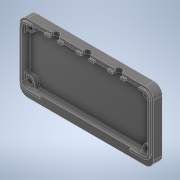
# Autodesk Inventor part: casing-bot
Saved by Autodesk Inventor 2021 (Build 250183000, 183)
## iProperties
Created: 2022-04-08
Part Number: casing-bot
Material: PET Plastic
Document SubType Name: Modeling
Designer: Staňa
Density: 1.541 g/cm^3
Appearance: Smooth - Black
Author: Staňa
Autodesk Inventor part; units mm, degrees
ref_plane "YZ Plane" through (0, 0, 0) normal (1, 0, 0) x (0, 1, 0)
ref_plane "XZ Plane" through (0, 0, 0) normal (0, 1, 0) x (-1, 0, 0)
sketch "Sketch1" plane through (0, 0, 0) normal (0, 0, 1) x (1, 0, 0)
  line L0 (-50, 17.455) -> (-50, -20) construction
  arc A0 (-46.75, 20.705) -> (-50, 17.455) centre (-46.7497, 17.4547) ccw construction
  arc A1 (-50, -20) -> (-46.75, -23.25) centre (-46.7497, -19.9997) ccw construction
  line L1 (-46.75, -23.25) -> (46.75, -23.25) construction
  arc A2 (46.75, -23.25) -> (50, -20) centre (46.7497, -19.9997) ccw construction
  line L2 (50, -20) -> (50, 17.455) construction
  arc A3 (50, 17.455) -> (46.75, 20.705) centre (46.7497, 17.4547) ccw construction
  line L3 (46.75, 20.705) -> (-46.75, 20.705) construction
  line L4 (-50.25, 17.4547) -> (-50.25, -19.9997)
  arc A4 (-50.25, -19.9997) -> (-46.7497, -23.5) centre (-46.7497, -19.9997) ccw
  line L5 (-46.7497, -23.5) -> (46.7497, -23.5)
  arc A5 (46.7497, -23.5) -> (50.25, -19.9997) centre (46.7497, -19.9997) ccw
  line L6 (50.25, -19.9997) -> (50.25, 17.4547)
  arc A6 (50.25, 17.4547) -> (46.7497, 20.955) centre (46.7497, 17.4547) ccw
  line L7 (46.7497, 20.955) -> (-46.7497, 20.955)
  arc A7 (-46.7497, 20.955) -> (-50.25, 17.4547) centre (-46.7497, 17.4547) ccw
  line L8 (-53.25, 17.7496) -> (-53.25, -23.7996)
  line L9 (53.25, -23.7996) -> (53.25, 17.7496)
  line L10 (46.7497, 24.2499) -> (-46.7497, 24.2499)
  line L11 (-32.1701, 24.2499) -> (-42.8301, 24.2499) construction
  line L12 (-2.2499, -30.2999) -> (-35.5799, -30.2999) construction
  arc A8 (-46.7497, 24.2499) -> (-53.25, 17.7496) centre (-46.7497, 17.7496) ccw
  arc A9 (53.25, 17.7496) -> (46.7497, 24.2499) centre (46.7497, 17.7496) ccw
  line L13 (-46.7497, -30.2999) -> (46.7497, -30.2999)
  arc A10 (-53.25, -23.7996) -> (-46.7497, -30.2999) centre (-46.7497, -23.7996) ccw
  arc A11 (46.7497, -30.2999) -> (53.25, -23.7996) centre (46.7497, -23.7996) ccw
  line L14 (-46.7497, 20.955) -> (-46.7497, 24.2499)
  line L15 (-46.7497, -23.5) -> (-46.7497, -30.2999)
  point P0 (0, 0)
  dimension "d0" = 0.25
  dimension "d1" = 3
  dimension "d2" = 3
  constraints: 22 end point, 16 point on circle, 8 centre point, 8 tangent, 2 collinear, 2 equal radius, 2 parallel, 2 vertical, 1 horizontal, 7 other
  measures "d0" radial gap between concentric circles of A0 A7
  measures "d1" distance between parallel lines of L4 L8
  measures "d2" distance between parallel lines of L6 L9
extrude "base" add sketch "Sketch1" against normal blind 5 contours L4 A4 L15 A10 L8 A8 L14 A7 | L14 L10 A9 L9 A11 L13 L15 L5 A5 L6 A6 L7
sketch "Sketch2" plane through (0, 0, -5) normal (0, 0, -1) x (-1, 0, 0)
  arc A0 (46.7497, -30.2999) -> (53.25, -23.7996) centre (46.7497, -23.7996) ccw projected
  line L0 (53.25, -23.7996) -> (53.25, 17.7496) projected
  arc A1 (53.25, 17.7496) -> (46.7497, 24.2499) centre (46.7497, 17.7496) ccw projected
  line L1 (46.7497, 24.2499) -> (-46.7497, 24.2499) projected
  arc A2 (-46.7497, 24.2499) -> (-53.25, 17.7496) centre (-46.7497, 17.7496) ccw projected
  line L2 (-53.25, 17.7496) -> (-53.25, -23.7996) projected
  arc A3 (-53.25, -23.7996) -> (-46.7497, -30.2999) centre (-46.7497, -23.7996) ccw projected
  line L3 (-46.7497, -30.2999) -> (46.7497, -30.2999) projected
  arc A4 (50.25, 17.4547) -> (46.7497, 20.955) centre (46.7497, 17.4547) ccw construction
  line L4 (50.25, 17.4547) -> (50.25, -19.9997) construction
  arc A5 (46.7497, -23.5) -> (50.25, -19.9997) centre (46.7497, -19.9997) ccw construction
  line L5 (46.7497, -23.5) -> (-46.7497, -23.5) construction
  arc A6 (-50.25, -19.9997) -> (-46.7497, -23.5) centre (-46.7497, -19.9997) ccw construction
  line L6 (-50.25, -19.9997) -> (-50.25, 17.4547) construction
  arc A7 (-46.7497, 20.955) -> (-50.25, 17.4547) centre (-46.7497, 17.4547) ccw construction
  line L7 (-46.7497, 20.955) -> (46.7497, 20.955) construction
  point P0 (0, 0)
extrude "floor" add sketch "Sketch2" along normal blind 2
sketch "Sketch5" plane through (0, 0, 0) normal (0, 0, 1) x (1, 0, 0)
  arc A0 (-53.25, -23.7996) -> (-46.7497, -30.2999) centre (-46.7497, -23.7996) ccw construction
  line L0 (-46.7497, -30.2999) -> (46.7497, -30.2999) construction
  arc A1 (46.7497, -30.2999) -> (53.25, -23.7996) centre (46.7497, -23.7996) ccw construction
  line L1 (53.25, -23.7996) -> (53.25, 17.7496) construction
  arc A2 (53.25, 17.7496) -> (46.7497, 24.2499) centre (46.7497, 17.7496) ccw construction
  line L2 (46.7497, 24.2499) -> (-46.7497, 24.2499) construction
  arc A3 (-46.7497, 24.2499) -> (-53.25, 17.7496) centre (-46.7497, 17.7496) ccw construction
  line L3 (-53.25, 17.7496) -> (-53.25, -23.7996) construction
  arc A4 (-46.7497, 20.955) -> (-50.25, 17.4547) centre (-46.7497, 17.4547) ccw projected
  line L4 (-46.7497, 20.955) -> (46.7497, 20.955) projected
  arc A5 (50.25, 17.4547) -> (46.7497, 20.955) centre (46.7497, 17.4547) ccw projected
  line L5 (50.25, 17.4547) -> (50.25, -19.9997) projected
  arc A6 (46.7497, -23.5) -> (50.25, -19.9997) centre (46.7497, -19.9997) ccw projected
  line L6 (46.7497, -23.5) -> (-46.7497, -23.5) projected
  arc A7 (-50.25, -19.9997) -> (-46.7497, -23.5) centre (-46.7497, -19.9997) ccw projected
  line L7 (-50.25, -19.9997) -> (-50.25, 17.4547) projected
  line L8 (42.8299, 15.7499) -> (42.8299, 24.2499) construction
  line L9 (32.1699, 24.2499) -> (32.1699, 15.7499) construction
  line L10 (17.8299, 15.7499) -> (17.8299, 24.2499) construction
  line L11 (7.1699, 24.2499) -> (7.1699, 15.7499) construction
  line L12 (-7.1701, 15.7499) -> (-7.1701, 24.2499) construction
  line L13 (-17.8301, 24.2499) -> (-17.8301, 15.7499) construction
  line L14 (-32.1701, 15.7499) -> (-32.1701, 24.2499) construction
  line L15 (-42.8301, 24.2499) -> (-42.8301, 15.7499) construction
  arc A8 (-46.7497, 22.455) -> (-51.75, 17.4547) centre (-46.7497, 17.4547) ccw
  arc A9 (51.75, 17.4547) -> (46.7497, 22.455) centre (46.7497, 17.4547) ccw
  line L16 (51.75, 17.4547) -> (51.75, -19.9997)
  arc A10 (46.7497, -25) -> (51.75, -19.9997) centre (46.7497, -19.9997) ccw
  arc A11 (-51.75, -19.9997) -> (-46.7497, -25) centre (-46.7497, -19.9997) ccw
  line L17 (-51.75, -19.9997) -> (-51.75, 17.4547)
  line L18 (-42.9801, 22.455) -> (-42.9801, 20.955)
  line L19 (-32.0201, 20.955) -> (-32.0201, 22.455)
  line L20 (-17.9801, 22.455) -> (-17.9801, 20.955)
  line L21 (-7.0201, 20.955) -> (-7.0201, 22.455)
  line L22 (7.0199, 22.455) -> (7.0199, 20.955)
  line L23 (17.9799, 20.955) -> (17.9799, 22.455)
  line L24 (32.0199, 22.455) -> (32.0199, 20.955)
  line L25 (42.9799, 20.955) -> (42.9799, 22.455)
  line L26 (42.9799, 22.455) -> (46.7497, 22.455)
  line L27 (17.9799, 22.455) -> (32.0199, 22.455)
  line L28 (-7.0201, 22.455) -> (7.0199, 22.455)
  line L29 (-46.7497, 22.455) -> (-42.9801, 22.455)
  line L30 (-32.0201, 22.455) -> (-17.9801, 22.455)
  line L31 (-46.7497, 20.955) -> (46.7497, 20.955) projected
  line L32 (-35.5799, -30.2999) -> (-35.5799, -21.4999) construction
  line L33 (35.5801, -21.4999) -> (35.5801, -30.2999) construction
  line L34 (35.7301, -23.5) -> (35.7301, -25)
  line L35 (-35.7299, -25) -> (-35.7299, -23.5)
  line L36 (46.7497, -25) -> (35.7301, -25)
  line L37 (-35.7299, -25) -> (-46.7497, -25)
  line L38 (46.7497, -23.5) -> (-46.7497, -23.5) construction
  point P0 (0, 0)
  point P1 (32.0199, 20.955)
  dimension "d36" = 1.5
  dimension "d37" = 0.15
  dimension "d38" = 0.15
  dimension "d39" = 0.15
  dimension "d40" = 0.15
  dimension "d41" = 0.15
  dimension "d42" = 0.15
  dimension "d43" = 0.15
  dimension "d44" = 0.15
  dimension "d52" = 0.15
  dimension "d53" = 0.15
  constraints: 40 end point, 24 point on line, 10 parallel, 8 point on circle, 5 collinear, 4 centre point, 4 tangent, 2 perpendicular, 6 other
  measures "d36" distance between parallel lines of L7 L17
  measures "d37" distance between parallel lines of L15 L18
  measures "d38" distance between parallel lines of L14 L19
  measures "d39" distance between parallel lines of L13 L20
  measures "d40" distance between parallel lines of L12 L21
  measures "d41" distance between parallel lines of L11 L22
  measures "d42" distance between parallel lines of L10 L23
  measures "d43" distance between parallel lines of L9 L24
  measures "d44" distance between parallel lines of L8 L25
  measures "d52" distance between parallel lines of L33 L34
  measures "d53" distance between parallel lines of L32 L35
extrude "top-indent" add sketch "Sketch5" along normal blind 1.5 contours A4 L7 A7 L6 L35 L37 A11 L17 A8 L29 L18 L4 | L19 L30 L20 L4 | L21 L28 L22 L4 | L6 A6 L5 A5 L4 L25 L26 A9 L16 A10 L36 L34 | L23 L27 L24 L4
sketch "Sketch6" plane through (-46.7497, 24.2499, 0) normal (-0.0000001, 1, 0) x (1, 0.0000001, 0)
  circle A0 centre (71.7497, -0.255) radius 3.25 construction
  arc A1 (69.0197, -1.7655) -> (69.0197, 1.2555) centre (71.7497, -0.255) ccw construction
  line L0 (69.0197, -1.7655) -> (69.0197, 1.2555) construction
  circle A2 centre (46.7497, -0.255) radius 3.25 construction
  arc A3 (44.0197, -1.7655) -> (44.0197, 1.2555) centre (46.7497, -0.255) ccw construction
  line L1 (44.0197, -1.7655) -> (44.0197, 1.2555) construction
  circle A4 centre (21.7497, -0.255) radius 3.25 construction
  arc A5 (19.0197, -1.7655) -> (19.0197, 1.2555) centre (21.7497, -0.255) ccw construction
  line L2 (19.0197, -1.7655) -> (19.0197, 1.2555) construction
  arc A6 (68.7697, -1.8287) -> (68.7697, 1.3187) centre (71.7497, -0.255) ccw
  line L3 (68.7697, -1.8287) -> (68.7697, 1.3187)
  arc A7 (43.7697, -1.8287) -> (43.7697, 1.3187) centre (46.7497, -0.255) ccw
  line L4 (43.7697, -1.8287) -> (43.7697, 1.3187)
  arc A8 (18.7697, -1.8287) -> (18.7697, 1.3187) centre (21.7497, -0.255) ccw
  line L5 (18.7697, -1.8287) -> (18.7697, 1.3187)
  line L6 (75.1197, -0.255) -> (75.1197, -3.625)
  line L7 (75.1197, -3.625) -> (71.7497, -3.625)
  line L8 (46.7497, -3.625) -> (50.1197, -3.625)
  line L9 (50.1197, -3.625) -> (50.1197, -0.255)
  line L10 (21.7497, -3.625) -> (25.1197, -3.625)
  line L11 (25.1197, -3.625) -> (25.1197, -0.255)
  point P0 (46.7497, 0)
  dimension "d47" = 0.25
  dimension "d48" = 0.25
  dimension "d49" = 0.25
  constraints: 18 end point, 12 point on circle, 6 tangent, 3 centre point, 3 perpendicular, 2 horizontal, 1 vertical, 3 other
  measures "d47" radial gap between concentric circles of A1 A6
  measures "d48" radial gap between concentric circles of A3 A7
  measures "d49" radial gap between concentric circles of A5 A8
extrude "coax-cutouts" cut sketch "Sketch6" against normal up to surface (3.2949 mm away)
sketch "Sketch7" plane through (0, 0, -5) normal (0, 0, 1) x (1, 0, 0)
  line L0 (46.7497, 20.955) -> (-46.7497, 20.955) projected
  arc A0 (-46.7497, 20.955) -> (-50.25, 17.4547) centre (-46.7497, 17.4547) ccw projected
  line L1 (-50.25, 17.4547) -> (-50.25, -19.9997) projected
  arc A1 (-50.25, -19.9997) -> (-46.7497, -23.5) centre (-46.7497, -19.9997) ccw projected
  line L2 (-46.7497, -23.5) -> (46.7497, -23.5) projected
  arc A2 (46.7497, -23.5) -> (50.25, -19.9997) centre (46.7497, -19.9997) ccw projected
  line L3 (50.25, -19.9997) -> (50.25, 17.4547) projected
  arc A3 (50.25, 17.4547) -> (46.7497, 20.955) centre (46.7497, 17.4547) ccw projected
  line L4 (0, 47.2668) -> (0, -42.6152) construction
  circle A4 centre (46.75, 17.455) radius 1.6 construction
  circle A5 centre (46.75, -20) radius 1.6 construction
  arc A6 (46.75, -16.5) -> (43.25, -20) centre (46.75, -20) ccw
  line L5 (46.75, -16.5) -> (48.35, -16.5)
  line L6 (50.25, -19.9997) -> (50.25, 17.4547) construction
  arc A7 (48.35, -16.5) -> (50.25, -14.6) centre (48.35, -14.6) ccw
  line L7 (48.35, -16.5) -> (48.35, -20) construction
  line L8 (43.25, -20) -> (43.25, -21.6)
  line L9 (43.25, -21.6) -> (46.75, -21.6) construction
  line L10 (-46.7497, -23.5) -> (46.7497, -23.5) projected
  arc A8 (41.35, -23.5) -> (43.25, -21.6) centre (41.35, -21.6) ccw
  arc A9 (43.25, 17.455) -> (46.75, 13.955) centre (46.75, 17.455) ccw
  line L11 (46.75, 13.955) -> (48.35, 13.955)
  line L12 (48.35, 13.955) -> (48.35, 17.455) construction
  line L13 (43.25, 17.455) -> (43.25, 19.055)
  line L14 (43.25, 19.055) -> (46.75, 19.055) construction
  line L15 (46.7497, 20.955) -> (-46.7497, 20.955) projected
  arc A10 (43.25, 19.055) -> (41.35, 20.955) centre (41.35, 19.055) ccw
  arc A11 (50.25, 12.055) -> (48.35, 13.955) centre (48.35, 12.055) ccw
  arc A12 (-43.25, -20) -> (-46.75, -16.5) centre (-46.75, -20) ccw
  line L16 (-46.75, -16.5) -> (-48.35, -16.5)
  arc A13 (-50.25, -14.6) -> (-48.35, -16.5) centre (-48.35, -14.6) ccw
  line L17 (-43.25, -20) -> (-43.25, -21.6)
  arc A14 (-43.25, -21.6) -> (-41.35, -23.5) centre (-41.35, -21.6) ccw
  arc A15 (-46.75, 13.955) -> (-43.25, 17.455) centre (-46.75, 17.455) ccw
  line L18 (-46.75, 13.955) -> (-48.35, 13.955)
  line L19 (-43.25, 17.455) -> (-43.25, 19.055)
  arc A16 (-41.35, 20.955) -> (-43.25, 19.055) centre (-41.35, 19.055) ccw
  arc A17 (-48.35, 13.955) -> (-50.25, 12.055) centre (-48.35, 12.055) ccw
  point P0 (0, 0)
  point P1 (-41.35, -23.5)
  point P2 (41.35, -23.5)
  dimension "d54" = 3.5
  constraints: 28 point on circle, 26 end point, 18 symmetric about line, 16 tangent, 12 centre point, 5 point on line, 4 vertical, 3 perpendicular, 2 coincident, 2 horizontal, 1 equal radius, 6 other
  measures "d54" radius of A6
ref_plane "Work Plane2" through (-50, -23.25, -1.6) normal (0, 0, -1) x (0, 1, 0)
extrude "pcb-support" add sketch "Sketch7" along normal up to surface (3.4 mm away) contours A3 L3 A11 L11 A9 L13 A10 L0 | A16 L19 A15 L18 A17 L1 A0 L0 | L3 A2 L2 A8 L8 A6 L5 A7 | A13 L16 A12 L17 A14 L2 A1 L1
fillet "pcb-support-fillet" radius 0.5 36 edges at (-47.55, 13.955, -5) (-49.6935, 13.3985, -5) (-50.25, -1.2725, -5) (-49.6935, -15.9435, -5) (-47.55, -16.5, -5) (-44.2751, -17.5251, -5) (-43.25, -20.8, -5) (-42.6935, -22.9435, -5) (0, -23.5, -5) (42.6935, -22.9435, -5) (43.25, -20.8, -5) (44.2751, -17.5251, -5) (47.55, -16.5, -5) (49.6935, -15.9435, -5) (50.25, -1.2725, -5) (49.6935, 13.3985, -5) (47.55, 13.955, -5) (44.2751, 14.9801, -5) (43.25, 18.255, -5) (42.6935, 20.3985, -5) (0, 20.955, -5) (-42.6935, 20.3985, -5) (-43.25, 18.255, -5) (-44.2751, 14.9801, -5) (-49.2248, 19.9298, -1.6) (-50.25, 14.7548, -1.6) (-44.0498, 20.955, -1.6) (-50.25, -17.2998, -1.6) (-44.0498, -23.5, -1.6) (-49.2248, -22.4748, -1.6) (50.25, 14.7548, -1.6) (44.0498, 20.955, -1.6) (49.2248, 19.9298, -1.6) (44.0498, -23.5, -1.6) (50.25, -17.2998, -1.6) (49.2248, -22.4748, -1.6)
sketch "Sketch8" plane through (41.35, -23.5, -1.6) normal (0, 0, 1) x (1, 0, 0)
  arc A0 (5.4, 7) -> (1.9, 3.5) centre (5.4, 3.5) ccw construction
  arc A1 (1.9, 40.955) -> (5.4, 37.455) centre (5.4, 40.955) ccw construction
  arc A2 (-88.1, 37.455) -> (-84.6, 40.955) centre (-88.1, 40.955) ccw construction
  arc A3 (-84.6, 3.5) -> (-88.1, 7) centre (-88.1, 3.5) ccw construction
  point P0 (-41.35, 23.5)
hole "insert-holes" at (46.75, -20, -1.6) at (46.75, 17.455, -1.6) at (-46.75, 17.455, -1.6) at (-46.75, -20, -1.6) direction (0, 0, -1) diameter 4.1 depth 4.3
equation "\"d2\" = d1"
equation "\"d38\" = d37"
equation "\"d39\" = d37"
equation "\"d40\" = d37"
equation "\"d41\" = d37"
equation "\"d42\" = d37"
equation "\"d43\" = d37"
equation "\"d44\" = d37"
equation "\"d52\" = d37"
equation "\"d53\" = d37"
body "Solid2"
